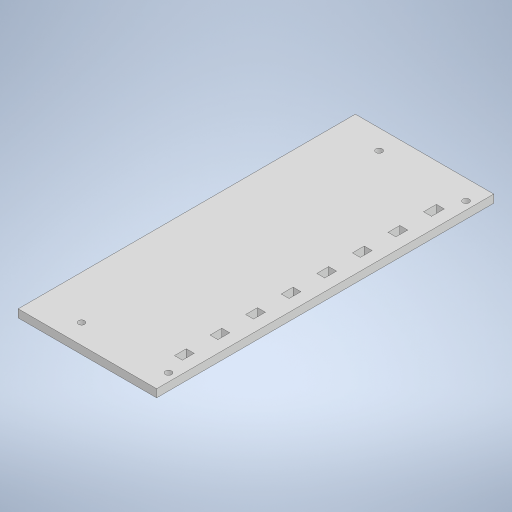
# Autodesk Inventor part: Деталь4
Saved by Autodesk Inventor 2023.1 (Build 271208000, 208)
## iProperties
Created: 2026-02-21
Part Number: Деталь4
Material: Типовые
Document SubType Name: Modeling
Designer: DELL
Density: 1 g/cm^3
Appearance: По умолчанию
Author: DELL
Autodesk Inventor part; units mm, degrees
ref_plane "YZ Plane" through (0, 0, 0) normal (1, 0, 0) x (0, 1, 0)
ref_plane "XZ Plane" through (0, 0, 0) normal (0, 1, 0) x (-1, 0, 0)
ref_plane "XY Plane" through (0, 0, 0) normal (0, 0, 1) x (1, 0, 0)
sketch "Эскиз1" plane through (0, 0, 0) normal (0, 1, 0) x (-1, 0, 0)
  line L0 (-35, 85.25) -> (35, 85.25)
  line L1 (35, 85.25) -> (35, -85.25)
  line L2 (35, -85.25) -> (-35, -85.25)
  line L3 (-35, -85.25) -> (-35, 85.25)
  line L4 (-35, 85.25) -> (35, -85.25) construction
  line L5 (35, 85.25) -> (-35, -85.25) construction
  circle A0 centre (13, 75.25) radius 1.6
  circle A1 centre (-31, 75.25) radius 1.6
  line L6 (35, 0) -> (0, 0) construction
  line L7 (-35, -85.25) -> (35, 85.25) construction
  circle A2 centre (13, -75.25) radius 1.6
  circle A3 centre (-31, -75.25) radius 1.6
  dimension "d0" = 170.5
  dimension "d1" = 70
  dimension "d2" = 3.2
  dimension "d3" = 22
  dimension "d4" = 10
  dimension "d5" = 3.2
  dimension "d6" = 4
  dimension "d7" = 10
  constraints: 16 end point, 4 centre point, 3 midpoint, 2 horizontal, 2 parallel, 2 symmetric about line, 1 perpendicular, 2 other
  measures "d0" distance of L2.end L0.start
  measures "d1" distance of L0.start L0.end
  measures "d2" diameter of A0
  measures "d3" distance from line of L1 A0.centre
  measures "d4" distance from line of L0 A0.centre
  measures "d5" diameter of A1
  measures "d6" distance from line of L3 A1.centre
  measures "d7" distance from line of L0 A1.centre
extrude "Выдавливание1" add sketch "Эскиз1" along normal blind 4
sketch "Эскиз2" plane through (0, 4, 0) normal (0, 1, 0) x (1, 0, 0)
  line L0 (29, -66.25) -> (25, -66.25) construction
  line L1 (25, 66.25) -> (29, 66.25) construction
  line L2 (29, 66.25) -> (29, -66.25) construction
  line L3 (35, -85.25) -> (35, 85.25) construction
  line L4 (-35, -85.25) -> (35, -85.25) projected
  line L5 (35, 85.25) -> (-35, 85.25) projected
  line L6 (25, -66.25) -> (29, -66.25)
  line L7 (29, -66.25) -> (29, -60.25)
  line L8 (29, -60.25) -> (25, -60.25)
  line L9 (25, -60.25) -> (25, -66.25)
  line L10 (25, -48.25) -> (29, -48.25)
  line L11 (25, -42.25) -> (25, -48.25)
  line L12 (29, -48.25) -> (29, -42.25)
  line L13 (29, -42.25) -> (25, -42.25)
  line L14 (25, -30.25) -> (29, -30.25)
  line L15 (25, -24.25) -> (25, -30.25)
  line L16 (29, -30.25) -> (29, -24.25)
  line L17 (29, -24.25) -> (25, -24.25)
  line L18 (25, -12.25) -> (29, -12.25)
  line L19 (25, -6.25) -> (25, -12.25)
  line L20 (29, -12.25) -> (29, -6.25)
  line L21 (29, -6.25) -> (25, -6.25)
  line L22 (25, 5.75) -> (29, 5.75)
  line L23 (25, 11.75) -> (25, 5.75)
  line L24 (29, 5.75) -> (29, 11.75)
  line L25 (29, 11.75) -> (25, 11.75)
  line L26 (25, 23.75) -> (29, 23.75)
  line L27 (25, 29.75) -> (25, 23.75)
  line L28 (29, 23.75) -> (29, 29.75)
  line L29 (29, 29.75) -> (25, 29.75)
  line L30 (25, 41.75) -> (29, 41.75)
  line L31 (25, 47.75) -> (25, 41.75)
  line L32 (29, 41.75) -> (29, 47.75)
  line L33 (29, 47.75) -> (25, 47.75)
  line L34 (29, 66.25) -> (25, 66.25)
  line L35 (25, 66.25) -> (25, 59.75)
  line L36 (25, 59.75) -> (29, 59.75)
  line L37 (29, 59.75) -> (29, 66.25)
  point P0 (27, -66.25)
  point P1 (27, 66.25)
  dimension "d12" = 4
  dimension "d13" = 6
  dimension "d14" = 19
  dimension "d15" = 19
  dimension "d16" = 4
  dimension "d17" = 6
  dimension "d20" = 18
  dimension "d25" = 4
  dimension "d26" = 6.5
  constraints: 70 end point, 5 parallel, 3 horizontal, 2 midpoint, 2 perpendicular, 1 vertical, 48 other
  measures "d12" distance of L1.start L1.end
  measures "d13" distance between parallel lines of L3 L2
  measures "d14" distance from line of L4 point (27, -66.25)
  measures "d15" distance from line of L5 point (27, 66.25)
  measures "d16" distance of L8.end L7.end
  measures "d17" distance of L7.end L6.end
  measures "d20" distance of L0.end L10.start
  measures "d25" distance of L35.end L36.end
  measures "d26" distance of L34.end L35.end
extrude "Выдавливание2" cut sketch "Эскиз2" against normal blind 10
